Autodesk Inventor part; units mm, degrees
(part 2 of 2)
  spline S227 degree 2 poles (-19.5253, -16.1642) (-19.2965, -16.2364) (-18.9642, -16.4149) (-18.7932, -16.614) knots 0 0 0 1 2 2 2
  spline S228 degree 2 poles (-18.7932, -16.614) (-18.6665, -16.7616) (-18.5108, -17.1041) (-18.4986, -17.2889) knots 0 0 0 1 2 2 2
  spline S229 degree 2 poles (-18.4986, -17.2889) (-18.4847, -17.5374) (-18.7016, -18.0289) (-18.9921, -18.2783) knots 0 0 0 1 2 2 2
  spline S230 degree 2 poles (-18.9921, -18.2783) (-19.2193, -18.4734) (-19.7339, -18.6466) (-19.9951, -18.6267) knots 0 0 0 1 2 2 2
  spline S231 degree 2 poles (-19.9951, -18.6267) (-20.2564, -18.6069) (-20.7656, -18.336) (-20.9808, -18.0854) knots 0 0 0 1 2 2 2
  spline S232 degree 2 poles (-20.9808, -18.0854) (-21.198, -17.8324) (-21.3934, -17.3205) (-21.3665, -17.0532) knots 0 0 0 1 2 2 2
  spline S233 degree 2 poles (-21.3665, -17.0532) (-21.3433, -16.7485) (-20.9681, -16.1333) (-20.5979, -15.8155) knots 0 0 0 1 2 2 2
  spline S234 degree 2 poles (-20.0882, -16.6272) (-20.3248, -16.8303) (-20.561, -17.1714) (-20.5829, -17.3165) knots 0 0 0 1 2 2 2
  spline S235 degree 2 poles (-20.5829, -17.3165) (-20.604, -17.42) (-20.5492, -17.5927) (-20.4869, -17.6653) knots 0 0 0 1 2 2 2
  spline S236 degree 2 poles (-20.4869, -17.6653) (-20.4306, -17.7309) (-20.2744, -17.8085) (-20.1606, -17.8084) knots 0 0 0 1 2 2 2
  spline S237 degree 2 poles (-20.1606, -17.8084) (-20.0621, -17.8093) (-19.7839, -17.6926) (-19.6551, -17.5819) knots 0 0 0 1 2 2 2
  spline S238 degree 2 poles (-19.6551, -17.5819) (-19.5145, -17.4613) (-19.3965, -17.2338) (-19.3949, -17.1266) knots 0 0 0 1 2 2 2
  spline S239 degree 2 poles (-19.3949, -17.1266) (-19.3953, -17.0171) (-19.4879, -16.8239) (-19.5724, -16.7255) knots 0 0 0 1 2 2 2
  spline S240 degree 2 poles (-19.5724, -16.7255) (-19.6428, -16.6436) (-19.8341, -16.5108) (-19.9038, -16.477) knots 0 0 0 1 2 2 2
  spline S241 degree 2 poles (-19.9038, -16.477) (-19.9249, -16.4951) (-20.0086, -16.5588) (-20.0882, -16.6272) knots 0 0 0 1 2 2 2
  dimension "d145" = 47.625
  constraints: 1 centre point, 1 coincident, 1 other
  measures "d145" diameter of A0
extrude "Extrusion19" cut sketch "Sketch26" against normal blind 1.905
equation "\"d103\" = hexDiameter"
equation "\"d110\" = centerLineForSpool"
equation "\"d111\" = centerLineForSpool"
equation "\"d112\" = holeForString"
equation "\"d121\" = centerLineForSpool"
equation "\"d122\" = holeForString"
equation "\"d125\" = knotHoleDiameter"
equation "\"d127\" = holeForString"
equation "\"d128\" = centerLineForSpool"
equation "\"d129\" = knotHoleDiameter"
equation "\"d130\" = knotHoleDepth"
equation "\"d86\" = spoolOverallHeight"
equation "\"d89\" = 0.5 * spoolOverallHeight"
equation "\"centerLineForSpool\" = 0.25 * spoolOverallHeight"
equation "\"holeForString\" = stringDiameter + clearanceForString"
equation "\"stringDiameter\" = 3.048"
equation "\"clearanceForString\" = 2.032"
equation "\"hexShaftDiameter\" = 12.7"
equation "\"clearanceForHexShaft\" = 1.016"
equation "\"hexDiameter\" = hexShaftDiameter + clearanceForHexShaft"
equation "\"spoolInteriorDiameter\" = 38.1"
equation "\"spoolInteriroRadius\" = 0.5 * spoolInteriorDiameter"
equation "\"spoolExteriorDiameter\" = 63.5"
equation "\"spoolExteriorRadius\" = 0.5 * spoolExteriorDiameter"
equation "\"hexHoleChamfer\" = 1.5875"
equation "\"stringHoleCenterFromHexShaft\" = 0.5 * hexDiameter + 0.5 * holeForString"
equation "\"textCircleDiameter\" = 0.75 * spoolExteriorDiameter"
equation "\"textHeight\" = 4.572"
equation "\"textDepth\" = 1.27"
equation "\"spoolOverallHeight\" = 69.85"
equation "\"d114\" = -spoolInteriroRadius"
equation "\"knotHoleDiameter\" = 9.525"
equation "\"d126\" = spoolInteriroRadius"
equation "\"metalWasherID\" = 26.67"
equation "\"metalWasherThickness\" = 0"
equation "\"spacerOD\" = 24.13"
equation "\"spacerThickness\" = 2.54"
equation "\"knotHoleDepth\" = 11.1125"
body "Solid3"
